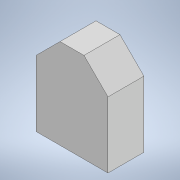
# Autodesk Inventor part: middle-join
Saved by Autodesk Inventor 2021 (Build 250183000, 183)
## iProperties
Created: 2020-12-10
Part Number: middle-join
Material: Generic
Document SubType Name: Modeling
Designer: Luke Kamols
Density: 1 g/cm^3
Appearance: Default
Author: Luke Kamols
Autodesk Inventor part; units mm, degrees
ref_plane "YZ Plane" through (0, 0, 0) normal (1, 0, 0) x (0, 1, 0)
ref_plane "XZ Plane" through (0, 0, 0) normal (0, 1, 0) x (-1, 0, 0)
ref_plane "XY Plane" through (0, 0, 0) normal (0, 0, 1) x (1, 0, 0)
sketch "Sketch1" plane through (0, 0, 0) normal (0, 0, 1) x (1, 0, 0)
  line L0 (0, 0) -> (6, 0)
  line L1 (6, 0) -> (6, 11)
  line L2 (0, 0) -> (-6, 0)
  line L3 (-6, 0) -> (-6, 11)
  line L4 (0, 0) -> (0, 15)
  line L5 (0, 15) -> (2, 15)
  line L6 (2, 15) -> (6, 11)
  line L7 (0, 15) -> (-2, 15)
  line L8 (-2, 15) -> (-6, 11)
  dimension "d0" = 6
  dimension "d1" = 11
  dimension "d2" = 6
  dimension "d3" = 11
  dimension "d4" = 15
  dimension "d5" = 2
  dimension "d6" = 2
  constraints: 18 end point, 4 perpendicular, 2 horizontal, 2 point on line, 1 vertical
  measures "d0" distance of L0.start L0.end
  measures "d1" distance of L0.end L1.end
  measures "d2" distance of L0.start L2.end
  measures "d3" distance of L2.end L3.end
  measures "d4" distance of L0.start L4.end
  measures "d5" distance of L4.end L5.end
  measures "d6" distance of L4.end L7.end
extrude "Extrusion1" add sketch "Sketch1" along normal blind 6
body "Solid1"
